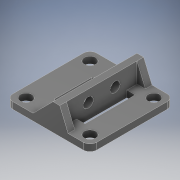
# Autodesk Inventor part: antennabrace
Saved by Autodesk Inventor 2022 (Build 260153000, 153)
## iProperties
Created: 2022-04-25
Part Number: antennabrace
Material: PBT Plastic
Document SubType Name: Modeling
Designer: Bowen
Density: 1.31 g/cm^3
Appearance: Smooth - Black
Author: Bowen
Autodesk Inventor part; units mm, degrees
ref_plane "YZ Plane" through (0, 0, 0) normal (1, 0, 0) x (0, 1, 0)
ref_plane "XZ Plane" through (0, 0, 0) normal (0, 1, 0) x (-1, 0, 0)
ref_plane "XY Plane" through (0, 0, 0) normal (0, 0, 1) x (1, 0, 0)
sketch "Sketch7" plane through (0, 0, 0) normal (1, 0, 0) x (0, 1, 0)
  line L0 (3.5, 10) -> (-3.5, 10)
  line L1 (-3.5, 10) -> (-3.5, -10)
  line L2 (-3.5, -10) -> (3.5, -10)
  line L3 (3.5, -10) -> (3.5, 10)
  point P0 (0, 0)
  point P1 (3.5, 0)
  point P2 (0, -10)
  dimension "d28" = 20
  dimension "d29" = 7
  constraints: 8 end point, 2 midpoint, 2 parallel, 1 horizontal, 1 horizontal alignment, 1 perpendicular, 1 vertical alignment
  measures "d28" distance of L1.end L0.end
  measures "d29" distance of L1.end L2.end
extrude "Extrusion5" add sketch "Sketch7" along normal mid plane 1
sketch "Sketch8" plane through (-0.5, -3.5, -10) normal (0, -1, 0) x (1, 0, 0)
  line L0 (-12.55, 22.55) -> (12.55, 22.55)
  line L1 (12.55, 22.55) -> (12.55, -2.55)
  line L2 (12.55, -2.55) -> (-12.55, -2.55)
  line L3 (-12.55, -2.55) -> (-12.55, 22.55)
  line L4 (0, 0) -> (0, 20) projected
  point P0 (0.5, 10)
  point P1 (12.55, 10)
  point P2 (0, 10)
  point P3 (0, 22.55)
  point P4 (0, 10)
  dimension "d32" = 25.1
  dimension "d33" = 25.1
  constraints: 8 end point, 4 midpoint, 2 parallel, 1 horizontal, 1 horizontal alignment, 1 perpendicular, 1 vertical alignment
  measures "d32" distance of L1.end L2.end
  measures "d33" distance of L0.end L1.end
extrude "Extrusion6" add sketch "Sketch8" along normal blind 1
sketch "Sketch9" plane through (-0.5, -3.5, -10) normal (0, 1, 0) x (1, 0, 0)
  line L0 (0, 0) -> (0, -20) projected
  line L1 (0, 0) -> (-5, 0)
  line L2 (-5, 0) -> (-5, -20)
  line L3 (-5, -20) -> (0, -20)
  line L4 (0, -20) -> (0, 0)
  point P0 (0.5, -10)
  dimension "d36" = 5
  dimension "d37" = 20
  constraints: 8 end point, 2 parallel, 1 horizontal, 1 perpendicular
  measures "d36" distance of L3.end L2.end
  measures "d37" distance of L2.end L1.end
extrude "Extrusion7" cut sketch "Sketch9" against normal through all
sketch "Sketch10" plane through (-0.5, 0, 0) normal (-1, 0, 0) x (0, 0, 1)
  point P0 (0, 0)
  point P1 (0, 0)
  constraints: 1 coincident
hole "Hole3" at (-0.5, 0, 0) direction (1, 0, 0) diameter 1.854 end through all clearance for "Flat Head Machine Screw (82)" size "#0" standard "Ansi Unified Screw Threads"
sketch "Sketch12" plane through (-0.5, -3.5, -10) normal (0, 1, 0) x (1, 0, 0)
  line L0 (12.55, 2.55) -> (12.55, -22.55) projected
  line L1 (-12.55, 2.55) -> (12.55, 2.55) projected
  line L2 (12.55, -10) -> (9.9413, -10) construction
  line L3 (-12.55, 2.55) -> (12.55, 2.55) construction
  line L4 (0, 2.55) -> (0, 1.0755) construction
  point P0 (0.5, -10)
  point P1 (9.55, -0.45)
  point P2 (9.55, -19.55)
  point P3 (-9.55, -0.45)
  point P4 (-9.55, -19.55)
  dimension "d53" = 3
  dimension "d54" = 3
  constraints: 4 end point, 3 symmetric about line, 2 midpoint, 1 horizontal, 1 vertical
  measures "d53" distance from line of L0 point (9.55, -0.45)
  measures "d54" distance from line of point (9.55, -0.45) L1
hole "Hole4" at (9.05, -3.5, -9.55) at (9.05, -3.5, 9.55) at (-10.05, -3.5, -9.55) at (-10.05, -3.5, 9.55) direction (0, -1, 0) diameter 3.454 end through all clearance for "Flat Head Machine Screw (82)" size "#4" standard "Ansi Unified Screw Threads"
sketch "Sketch13" plane through (0.5, 0, 0) normal (1, 0, 0) x (0, 0, -1)
  line L0 (-10, -3.5) -> (10, -3.5) projected
  line L1 (10, -3.5) -> (10, 3.5) projected
  line L2 (10, 3.5) -> (-10, 3.5) projected
  line L3 (-10, 3.5) -> (-10, -3.5) projected
  point P0 (0, 0)
extrude "Extrusion9" add sketch "Sketch13" along normal blind 2.5
sketch "Sketch14" plane through (-0.5, 0, 0) normal (-1, 0, 0) x (0, 0, 1)
  line L0 (10, -3.5) -> (10, 3.5) projected
  line L1 (10, 3.5) -> (-10, 3.5) projected
  line L2 (-10, 3.5) -> (-10, -3.5) projected
  line L3 (-10, -3.5) -> (-10, -4.5) projected
  line L4 (10, -4.5) -> (-10, -4.5) projected
  line L5 (10, -3.5) -> (10, -4.5) projected
  point P0 (0, 0)
extrude "Extrusion10" cut sketch "Sketch14" against normal blind 1.5
sketch "Sketch15" plane through (-0.5, -3.5, -10) normal (0, 1, 0) x (1, 0, 0)
  line L0 (12.55, 2.55) -> (12.55, -22.55) projected
  line L1 (12.55, -22.55) -> (-12.55, -22.55) projected
  line L2 (12.55, 2.55) -> (-12.55, 2.55)
  line L3 (-12.55, 2.55) -> (-12.55, -22.55)
  line L4 (-12.55, -22.55) -> (12.55, -22.55)
  line L5 (12.55, -22.55) -> (12.55, 2.55)
  circle A0 centre (0, -10) radius 7.5
  circle A1 centre (-9.55, -0.45) radius 1.727 projected
  circle A2 centre (-9.55, -19.55) radius 1.727 projected
  circle A3 centre (9.55, -19.55) radius 1.727 projected
  circle A4 centre (9.55, -0.45) radius 1.727 projected
  point P0 (0.5, -10)
  point P1 (0, -22.55)
  point P2 (12.55, -10)
  dimension "d66" = 15
  constraints: 8 end point, 2 midpoint, 2 parallel, 1 centre point, 1 horizontal, 1 horizontal alignment, 1 perpendicular, 1 vertical alignment
  measures "d66" diameter of A0
extrude "Extrusion11" add sketch "Sketch15" against normal up to surface (1 mm away)
sketch "Sketch16" plane through (-0.5, -3.5, -10) normal (0, 1, 0) x (1, 0, 0)
  line L0 (6, -2.5) -> (3.5, -2.5)
  line L1 (3.5, -2.5) -> (3.5, -17.5)
  line L2 (3.5, -17.5) -> (6, -17.5)
  line L3 (6, -17.5) -> (6, -2.5)
  line L4 (3.5, 0) -> (3.5, -20) projected
  point P0 (0.5, -10)
  point P1 (3.5, -10)
  point P2 (3.5, -10)
  point P3 (3.5, -10)
  dimension "d69" = 15
  dimension "d70" = 2.5
  constraints: 8 end point, 4 midpoint, 2 parallel, 1 coincident, 1 horizontal, 1 perpendicular
  measures "d69" distance of L2.end L0.start
  measures "d70" distance of L1.end L2.end
extrude "Extrusion12" cut sketch "Sketch16" against normal through all
sketch "Sketch17" plane through (3, -3.5, -10) normal (0, 0, -1) x (-1, 0, 0)
  line L0 (2, 0) -> (2, 7) projected
  line L1 (2, 7) -> (0, 7) projected
  line L2 (0, 0) -> (0, 7) projected
  line L3 (2, 0) -> (0, 0) projected
  line L4 (16.05, 0) -> (-9.05, 0) projected
  line L5 (-9.05, 0) -> (-9.05, -1) projected
  line L6 (16.05, -1) -> (-9.05, -1) projected
  line L7 (16.05, 0) -> (16.05, -1) projected
  line L8 (2, 7) -> (9, 0)
  point P0 (3, 3.5)
  dimension "d73" = 7
  constraints: 2 end point, 1 point on line
  measures "d73" distance from line of L0 L8.end
extrude "Extrusion13" add sketch "Sketch17" along normal up to surface (2.55 mm away) contours L3 L2 L1 L0 | L0 L8 L4
sketch "Sketch18" plane through (3, -3.5, 10) normal (0, 0, 1) x (1, 0, 0)
  line L0 (-2, 0) -> (-2, 7) projected
  line L1 (-9, 0) -> (-2, 7) projected
  line L2 (-2, 0) -> (-9, 0) projected
  line L3 (-2, 7) -> (-2, 0) projected
  line L4 (0, 0) -> (-2, 0) projected
  line L5 (0, 7) -> (0, 0) projected
  line L6 (-2, 7) -> (0, 7) projected
  point P0 (-3, 3.5)
extrude "Extrusion14" add sketch "Sketch18" along normal up to surface (2.55 mm away)
fillet "Fillet1" radius 2 4 edges at (-13.05, -4, -12.55) (-13.05, -4, 12.55) (12.05, -4, 12.55) (12.05, -4, -12.55)
sketch "Sketch19" plane through (-0.5, -3.5, -10) normal (0, 1, 0) x (1, 0, 0)
  arc A0 (-12.55, -20.55) -> (-10.55, -22.55) centre (-10.55, -20.55) ccw projected
  line L0 (-5.5, -22.55) -> (-10.55, -22.55) projected
  line L1 (-5.5, -22.55) -> (-5.5, -20) projected
  line L2 (-5.5, -20) -> (1.5, -20) projected
  line L3 (1.5, -17.3485) -> (1.5, -20) projected
  arc A1 (-5, -15.5902) -> (1.5, -17.3485) centre (0, -10) ccw projected
  line L4 (-5, -15.5902) -> (-5, -4.4098) projected
  arc A2 (1.5, -2.6515) -> (-5, -4.4098) centre (0, -10) ccw projected
  line L5 (1.5, 0) -> (1.5, -2.6515) projected
  line L6 (1.5, 0) -> (-5.5, 0) projected
  line L7 (-5.5, 0) -> (-5.5, 2.55) projected
  line L8 (-10.55, 2.55) -> (-5.5, 2.55) projected
  arc A3 (-10.55, 2.55) -> (-12.55, 0.55) centre (-10.55, 0.55) ccw projected
  line L9 (-12.55, -20.55) -> (-12.55, 0.55) projected
  circle A4 centre (-9.55, -19.55) radius 1.727 projected
  circle A5 centre (-9.55, -0.45) radius 1.727 projected
  line L10 (1.5, 0) -> (-5.5, 0) projected
  line L11 (1.5, 0) -> (-0.5, 0)
  line L12 (-0.5, 0) -> (-0.5, -20)
  line L13 (-5.5, -20) -> (1.5, -20) projected
  arc A6 (12.55, 0.55) -> (10.55, 2.55) centre (10.55, 0.55) ccw projected
  line L14 (3.5, 2.55) -> (10.55, 2.55) projected
  line L15 (3.5, 2.55) -> (3.5, -2.5) projected
  line L16 (3.5, -2.5) -> (6, -2.5) projected
  line L17 (6, -2.5) -> (6, -17.5) projected
  line L18 (6, -17.5) -> (3.5, -17.5) projected
  line L19 (3.5, -17.5) -> (3.5, -22.55) projected
  line L20 (10.55, -22.55) -> (3.5, -22.55) projected
  arc A7 (10.55, -22.55) -> (12.55, -20.55) centre (10.55, -20.55) ccw projected
  line L21 (12.55, 0.55) -> (12.55, -20.55) projected
  circle A8 centre (9.55, -0.45) radius 1.727 projected
  circle A9 centre (9.55, -19.55) radius 1.727 projected
  line L22 (-5.5, 0) -> (-5.5, 2.55) projected
  line L23 (-5.5, 2.55) -> (-2.6367, 2.55)
  line L24 (-10.55, 2.55) -> (10.55, 2.55) projected
  line L25 (-5.5, -22.55) -> (1.5, -22.55) projected
  line L26 (-5.5, -22.55) -> (-2.6367, -22.55)
  line L27 (-2.6367, 2.55) -> (-2.6367, 0)
  line L28 (-2.6367, -22.55) -> (-2.6367, -20)
  point P0 (0.5, -10)
  point P1 (-0.5, -17.4833)
  point P2 (-0.5, -2.5167)
  dimension "d81" = 2
  constraints: 12 end point, 6 point on line, 3 perpendicular
  measures "d81" distance of L5.start L11.end
extrude "Extrusion15" add sketch "Sketch19" along normal blind 1 contours L9 A3 L8 L7 L6 L12 A2 L4 A1 L2 L1 L0 A0 | L1 L2 L28 L25 | L23 L27 L6 L7 | L21 A7 L20 L19 L18 L17 L16 L15 L14 A6
sketch "Sketch20" plane through (1, 0, 0) normal (-1, 0, 0) x (0, 0, 1)
  line L0 (0, 0) -> (-4, 0) construction
  line L1 (0, -1.5) -> (0, 1.5) construction
  line L2 (10.55, -2.5) -> (-10.55, -2.5) projected
  line L3 (-4, 0) -> (-4, 0) construction
  circle A0 centre (-4, 0) radius 1.5
  circle A1 centre (4, 0) radius 1.5
  dimension "d84" = 4
  dimension "d88" = 0
  dimension "d89" = 3
  constraints: 6 end point, 2 centre point, 2 vertical, 1 coincident, 1 horizontal, 1 symmetric about line, 1 other
  measures "d84" distance of L0.start L0.end
  measures "d88" distance of L0.end L3.end
  measures "d89" diameter of A0
extrude "Extrusion17" cut sketch "Sketch20" against normal up to surface (2 mm away)
sketch "Sketch21" plane through (3, 3.5, -12.55) normal (0, 0, -1) x (-1, 0, 0)
  line L0 (2, 0) -> (0, 0) projected
  line L1 (-2.5, -6) -> (-2.5, -8) projected
  line L2 (0, 0) -> (-2.5, -6)
  line L3 (0, -6) -> (0, -8) projected
  line L4 (-2.5, -6) -> (0, -6)
  line L5 (0, -6) -> (0, 0)
  point P0 (3, -3.5)
  constraints: 6 end point, 1 horizontal, 1 perpendicular
extrude "Extrusion18" add sketch "Sketch21" against normal blind 2
mirror "Mirror1" about plane through (0, 0, 0) normal (0, 0, 1) of "Extrusion18"
body "Solid2"
